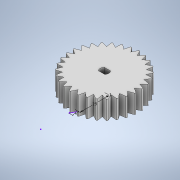
# Autodesk Inventor part: motor driven gear straight teeth
Saved by Autodesk Inventor 2022 (Build 260153000, 153)
## iProperties
Created: 2021-11-09
Part Number: motor driven gear straight teeth
Material: Generic
Document SubType Name: Modeling
Designer: a-dubs
Density: 1 g/cm^3
Appearance: Default
Author: a-dubs
Autodesk Inventor part; units mm, degrees
ref_plane "YZ Plane" through (0, 0, 0) normal (1, 0, 0) x (0, 1, 0)
ref_plane "XZ Plane" through (0, 0, 0) normal (0, 1, 0) x (-1, 0, 0)
ref_plane "XY Plane" through (0, 0, 0) normal (0, 0, 1) x (1, 0, 0)
sketch "Sketch1" plane through (0, 0, 0) normal (0, 1, 0) x (-1, 0, 0)
  line L0 (-2, 0) -> (2, 0)
  line L1 (-2, 0) -> (-2, 1)
  line L2 (-2, 1) -> (0, 0)
  line L3 (0, 0) -> (2, 1)
  line L4 (0, 0) -> (0, 19)
  line L5 (0, 19) -> (2, 19)
  line L6 (-2, 19) -> (0, 19)
  line L7 (0, 19) -> (0, 23)
  line L8 (0, 23) -> (-2, 19)
  line L9 (2, 19) -> (0, 23)
  line L10 (2, 0) -> (2, 19)
  line L11 (-2, 19) -> (-2, 0)
  point P0 (0, 41)
  dimension "d6" = 1
  dimension "d10" = 19
  dimension "d11" = 4
  constraints: 24 end point, 2 equal length, 1 vertical
  measures "d6" distance of L0.start L1.end
  measures "d10" distance of L2.end L4.end
  measures "d11" distance of L4.end L7.end
extrude "Extrusion1" add sketch "Sketch1" along normal blind 12 contours L3 L10 L0 | L4 L5 L10 L3 | L2 L11 L6 L4 | L7 L9 L5 | L6 L8 L7
pattern_circular "Circular Pattern1" count 30 over 360 about axis through (0, 0, 0) along (0, 1, 0) of "Extrusion1"
fillet "Fillet1" radius 0.5 1 edges at (0, 6, 23)
sketch "Sketch2" plane through (0, 12, 0) normal (0, 1, 0) x (1, 0, 0)
  circle A0 centre (0, 0) radius 1.5
  circle A1 centre (0, 0) radius 2.8
  line L0 (0, 0) -> (0, 1.9)
  line L1 (0, 1.9) -> (0, -1.9)
  line L2 (0, -1.9) -> (-2.0567, -1.9)
  line L3 (0, -1.9) -> (2.0567, -1.9)
  line L4 (0, 1.9) -> (2.0567, 1.9)
  line L5 (0, 1.9) -> (-2.0567, 1.9)
  dimension "d13" = 3
  dimension "d19" = 5.6
  dimension "d20" = 1.9
  dimension "d21" = 3.8
  constraints: 12 end point, 4 point on circle, 2 centre point, 2 coincident, 2 point on line, 1 parallel, 1 perpendicular, 1 vertical
  measures "d13" diameter of A0
  measures "d19" diameter of A1
  measures "d20" distance of L0.start L0.end
  measures "d21" distance of L0.end L1.end
extrude "Extrusion2" cut sketch "Sketch2" against normal blind 10 contours A0 L1 L0 | A0 L0 L4 A1 L3 L1 | L0 L1 A0 | A0 L1 L2 A1 L5 L0
pattern_circular "Circular Pattern2" count 30 over 360 about axis through (0, 12, 0) along (0, -1, 0) of "Fillet1"
extrude "Extrusion3" cut sketch "Sketch2" against normal blind 8 from surface at -10
chamfer "Chamfer1" distance 0.85 angle 45 2 edges at (0, 2, 1.9) (0, 2, -1.9)
body "Solid1"
